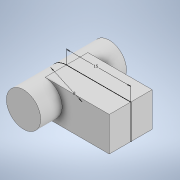
# Autodesk Inventor part: Pitch and Yaw
Saved by Autodesk Inventor 2020 (Build 240168000, 168)
## iProperties
Created: 2020-12-23
Part Number: Pitch and Yaw
Material: Generic
Document SubType Name: Modeling
Designer: frost
Density: 1 g/cm^3
Appearance: Default
Author: frost
Autodesk Inventor part; units mm, degrees
ref_plane "YZ Plane" through (0, 0, 0) normal (1, 0, 0) x (0, 1, 0)
ref_plane "XZ Plane" through (0, 0, 0) normal (0, 1, 0) x (-1, 0, 0)
ref_plane "XY Plane" through (0, 0, 0) normal (0, 0, 1) x (1, 0, 0)
sketch "Sketch1" plane through (0, 0, 0) normal (0, 0, 1) x (1, 0, 0)
  circle A0 centre (0, 0) radius 4
  line L0 (15, 1) -> (15, 4)
  line L1 (4, 0) -> (7.8423, 0)
  line L2 (15, 4) -> (0, 4)
  line L3 (15, -1) -> (15, -4)
  line L4 (15, -4) -> (0, -4)
  line L5 (15, 1) -> (15, -1)
  point P0 (0, -4)
  dimension "d0" = 8
  dimension "d2" = 15
  constraints: 12 end point, 3 symmetric about line, 2 point on circle, 2 vertical, 1 centre point, 1 coincident, 1 horizontal, 1 parallel, 1 tangent
  measures "d0" diameter of A0
  measures "d2" distance of L0.end L2.end
extrude "Extrusion1" add sketch "Sketch1" along normal mid plane 10 contours A0 L2 L0 L5 L3 L4
extrude "Extrusion2" add sketch "Sketch1" along normal mid plane 20 contours A0
body "Solid1"
